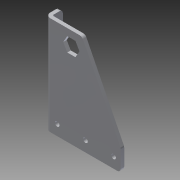
# Autodesk Inventor part: Spacer 3 (L-L) ipt
Saved by Autodesk Inventor 2014 (Build 180170000, 170)
## iProperties
Created: 2014-01-17
Part Number: Spacer 3 (L-L) ipt
Material: Aluminum 6061
Document SubType Name: Sheet Metal
Designer: Michael
Density: 2.71 g/cm^3
Sheet Metal Rule: Default
Appearance: Aluminum - Flat
Mass: 26.9463 g
Surface Area: 72.5808 cm^2
Volume: 9.94327 cm^3
Flat Pattern Width: 7.59443 cm
Flat Pattern Length: 8.89 cm
Flat Pattern Area: 67.5145 cm^2
Sheet Metal Width: 2.990 in
Sheet Metal Length: 3.500 in
Sheet Metal Area: 10.465 in^2
Author: Michael
Autodesk Inventor part; units mm, degrees
ref_plane "YZ Plane" through (0, 0, 0) normal (1, 0, 0) x (0, 1, 0)
ref_plane "XZ Plane" through (0, 0, 0) normal (0, 1, 0) x (-1, 0, 0)
ref_plane "XY Plane" through (0, 0, 0) normal (0, 0, 1) x (1, 0, 0)
sketch "Sketch1" plane through (0, 0, 0) normal (0, 0, 1) x (1, 0, 0)
  line L0 (0, 0) -> (63.5, 0)
  line L1 (63.5, 0) -> (63.5, 19.05)
  line L2 (0, 88.9) -> (0, 0)
  circle A0 centre (6.35, 9.525) radius 2.0701
  circle A1 centre (31.75, 9.525) radius 2.0701
  circle A2 centre (57.15, 9.525) radius 2.0701
  line L3 (63.5, 19.05) -> (28.575, 88.9)
  line L4 (28.575, 88.9) -> (0, 88.9)
  line L5 (22.7162, 82.55) -> (26.3823, 76.2)
  line L6 (26.3823, 76.2) -> (22.7162, 69.85)
  line L7 (22.7162, 69.85) -> (15.3838, 69.85)
  line L8 (15.3838, 69.85) -> (11.7177, 76.2)
  line L9 (11.7177, 76.2) -> (15.3838, 82.55)
  line L10 (15.3838, 82.55) -> (22.7162, 82.55)
  point P0 (19.05, 76.2)
  dimension "d5" = 63.5
  dimension "d6" = 4.1402
  dimension "d7" = 6.35
  dimension "d8" = 9.525
  dimension "d24" = 25.4
  dimension "d29" = 88.9
  dimension "d30" = 19.05
  dimension "d31" = 28.575
  dimension "d32" = 12.7
  dimension "d34" = 19.05
  dimension "d35" = 12.7
extrude "Plate1" add sketch "Sketch1" along normal blind 3.175
sketch "Sketch3" plane through (-1.27, 88.9, -1.27) normal (-1, 0, 0) x (0, -1, 0)
  line L0 (88.9, 0) -> (0, 0)
  line L1 (0, 0) -> (0, -8.255)
  line L2 (0, -8.255) -> (88.9, -8.255)
  line L3 (88.9, -8.255) -> (88.9, 0)
  constraints: 6 end point, 1 horizontal, 1 perpendicular, 1 vertical
edge flange "Flange2" height 12.7 angle 90 thickness 3.175 bend radius 1.27 thickness toward (-1, 0, 0) relief straight relief width 3.175 relief depth 1.5875 edges at (0, 44.45, 0) wall of the first edge with corners at (-1.27, 0, -1.27) (-1.27, 88.9, -1.27) (-1.27, 88.9, -9.525) (-1.27, 0, -9.525)
bend "Bend2"
corner "Corner2"
fillet "Fillet1" radius 3.175 5 edges at (28.575, 88.9, 1.5875) (-2.8575, 88.9, -9.525) (63.5, 19.05, 1.5875) (63.5, 0, 1.5875) (-2.8575, 0, -9.525)
equation "\"d36\" = BendReliefWidth"
equation "\"d37\" = BendReliefDepth"
equation "\"d38\" = MinimumRemnant"
equation "\"d39\" = BendRadius"
equation "\"d43\" = CornerReliefSize"
equation "\"d44\" = GapSize"
equation "\"d45\" = JacobiRadiusSize"
equation "\"BendRadius\" = Thickness"
equation "\"BendReliefWidth\" = Thickness"
equation "\"BendReliefDepth\" = 0.5 * Thickness"
equation "\"CornerReliefSize\" = 4 * Thickness"
equation "\"MinimumRemnant\" = 2 * Thickness"
equation "\"TransitionRadius\" = BendRadius"
equation "\"JacobiRadiusSize\" = BendRadius"
equation "\"GapSize\" = Thickness"
equation "\"d11\" = BendRadius"
equation "\"Thickness\" = 3.175"
body "Solid1"
